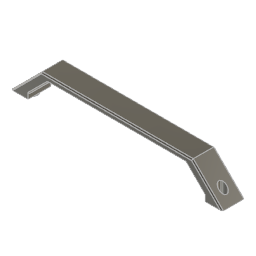
Drip tray handle (Autodesk Fusion 360 design; units mm, degrees)
Autodesk Fusion 360 part; units mm, degrees
mesh "Mesh1" [no effect]
sketch "Sketch1" plane through (0, -18.5, 0) normal (0, 1, 0) x (-1, 0, 0)
  line L0 (89, 54.6) -> (-89, 54.6)
  line L1 (-89, 54.6) -> (-89, 50)
  line L2 (-89, 50) -> (89, 50)
  line L3 (89, 50) -> (89, 54.6)
  line L4 (-69.8278, 56) -> (-74.5256, 56)
  line L5 (-87.6, 56) -> (-62.6, 81)
  line L6 (-87.6, 56) -> (-45.4555, 56) construction
  line L7 (-62.6, 81) -> (62.6, 81)
  line L8 (87.6, 56) -> (-87.6, 56)
  line L9 (0, 56) -> (0, 70)
  line L10 (-56.9934, 76) -> (56.9934, 76)
  line L11 (-76.9934, 56) -> (-56.9934, 76)
  line L12 (-73.3, 56) -> (-73.3, 70.3)
  line L13 (-73.3, 63.2) -> (-80.5, 56)
  line L14 (76.9934, 56) -> (56.9934, 76)
  line L15 (73.3, 63.2) -> (80.5, 56)
  line L16 (87.6, 56) -> (62.6, 81)
  line L17 (73.3, 56) -> (73.3, 70.3)
  dimension "d1" = 45
  dimension "d2" = 25
  dimension "d5" = 5
  constraint horizontal L6
  constraint coincident L5.start L6.start
  constraint horizontal L7
  constraint midpoint L8 L9.start
  constraint perpendicular L8 L9
  constraint symmetric L9 L5.end L7.end
  constraint parallel L5 L11
  constraint coincident L6 L11.start
  constraint symmetric L9 L10.start L10.end
  constraint parallel L7 L10
  constraint coincident L5 L12.end
  constraint perpendicular L8 L12
  constraint coincident L4 L12.start
  constraint coincident L12 L13.start
  constraint symmetric L5.start L9 L8.start
  constraint symmetric L9 L11.start L14.start
  constraint symmetric L9 L12.end L17.end
  constraint symmetric L9 L13.start L15.start
  constraint symmetric L9 L13.end L15.end
  constraint symmetric L9 L12.start L17.start
  measures "d1" angle of L5 L6
  measures "d2" distance of L7 L8
  measures "d5" distance of L7 L10
extrude "Extrude1" add sketch "Sketch1" against normal blind 19 contours L5 L7 L10 L11 L12 L14 L16 L17 | L8 L11 L12 L13 | L5 L8 L12 L13 | L8 L14 L15 L17 | L8 L15 L16 L17
chamfer "Chamfer2" distance 1 angle 45 12 edges at (66.9934, -18.5, 66) (0, -18.5, 76) (-66.9934, -18.5, 66) (-66.9934, -37.5, 66) (0, -37.5, 76) (66.9934, -37.5, 66) (75.1, -18.5, 68.5) (0, -18.5, 81) (-75.1, -18.5, 68.5) (-75.1, -37.5, 68.5) (0, -37.5, 81) (75.1, -37.5, 68.5)
extrude "Extrude2" add sketch "Sketch1" against normal blind 19 contours L4 L8 L11 L12 | L8 L11 L12 L13 | L8 L14 L17 | L8 L14 L15 L17
sketch "Sketch2" plane through (0, 0, 56) normal (0, 0, 1) x (-1, 0, 0)
  arc A0 (-69.8278, 79.6561) -> (-72.2713, 77.9446) centre (-69.8278, 77.0561) ccw
  line L0 (-69.8278, 79.6561) -> (69.8278, 79.6561)
  arc A1 (72.271, 77.9454) -> (69.8278, 79.6561) centre (69.8278, 77.0561) ccw
  line L1 (72.271, 77.9454) -> (85.5724, 41.4)
  line L2 (85.5724, 41.4) -> (-85.5724, 41.4)
  line L3 (-85.5724, 41.4) -> (-72.2713, 77.9446)
  line L4 (87.6, 19.9) -> (87.6, 42.8465)
  line L5 (87.6, 42.8465) -> (74.5263, 78.7662)
  arc A2 (74.5263, 78.7662) -> (69.8278, 82.0561) centre (69.8278, 77.0561) ccw
  line L6 (69.8278, 82.0561) -> (-69.8278, 82.0561)
  arc A3 (-69.8278, 82.0561) -> (-74.5256, 78.7681) centre (-69.8278, 77.0561) ccw
  line L7 (-74.5256, 78.7681) -> (-87.6, 42.8465)
  line L8 (-87.6, 42.8465) -> (-87.6, 19.9)
  line L9 (-87.6, 19.9) -> (87.6, 19.9)
  circle A4 centre (-79, 28.5) radius 5
  circle A5 centre (-79, 28.5) radius 3.25
  line L10 (0, 18.5) -> (0, 36.7248)
  circle A6 centre (79, 28.5) radius 3.25
  circle A7 centre (79, 28.5) radius 5
  circle A8 centre (-79, 28.5) radius 1.75
  circle A9 centre (79, 28.5) radius 1.75
  circle A10 centre (-79, 28.5) radius 5
  circle A11 centre (79, 28.5) radius 5
  point P0 (0, 18.5)
  dimension "d12" = 6.5
  dimension "d13" = 10
  dimension "d14" = 3.5
  constraint coincident P0 L10.start
  constraint perpendicular L9 L10
  constraint symmetric A4 L10 A7
  constraint symmetric A5 L10 A6
  constraint symmetric L10 A8 A9
  measures "d12" diameter of A5
  measures "d13" diameter of A4
  measures "d14" diameter of A8
extrude "Extrude3" cut sketch "Sketch2" along normal blind 20 from surface at 0.5 contours A5 | A6
extrude "Extrude4" add sketch "Sketch2" against normal blind 2 draft -5 contours A4 A10 | A5 | A6 | A7 A11
extrude "Extrude5" cut sketch "Sketch2" along normal mid plane 82 contours A8 | A9
